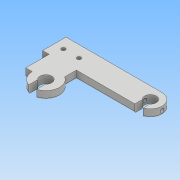
# Autodesk Inventor part: Hand - Digit 0-1
Saved by Autodesk Inventor 2017 (Build 210142000, 142)
## iProperties
Created: 2016-09-27
Part Number: Hand - Digit 0-1
Material: Generic
Document SubType Name: Modeling
Designer: cmcdona
Density: 1 g/cm^3
Appearance: Default
Author: cmcdona
Autodesk Inventor part; units mm, degrees
ref_plane "YZ Plane" through (0, 0, 0) normal (1, 0, 0) x (0, 1, 0)
ref_plane "XZ Plane" through (0, 0, 0) normal (0, 1, 0) x (-1, 0, 0)
sketch "Sketch1" plane through (0, 0, 0) normal (0, 0, 1) x (1, 0, 0)
  line L0 (0, 0) -> (5, 0)
  line L1 (5, 0) -> (5, -18)
  line L2 (5, -18) -> (26, -18)
  line L3 (26, -18) -> (26, 0)
  line L4 (26, 0) -> (74, 0)
  arc A0 (74, 0) -> (74, 18) centre (74, 9) ccw
  line L5 (74, 18) -> (0, 18)
  line L6 (0, 18) -> (0, 0)
  circle A1 centre (20.5, -18) radius 10.5
  dimension "d0" = 5
  dimension "d1" = 18
  dimension "d2" = 21
  dimension "d3" = 18
  dimension "d4" = 48
  dimension "d5" = 18
  dimension "d6" = 9
  dimension "d7" = 74
  dimension "d8" = 21
  constraints: 14 end point, 3 perpendicular, 3 point on line, 2 centre point, 2 horizontal, 2 point on circle
  measures "d0" distance of L0.start L0.end
  measures "d1" distance of L0.end L1.end
  measures "d2" distance of L1.end L2.end
  measures "d3" distance of L2.end L3.end
  measures "d4" distance of L3.end L4.end
  measures "d5" distance of L4.end L5.start
  measures "d6" radius of A0
  measures "d7" distance of L5.start L5.end
  measures "d8" diameter of A1
extrude "Extrusion1" add sketch "Sketch1" along normal blind 6
sketch "Sketch2" plane through (0, 0, 0) normal (0, 0, -1) x (-1, 0, 0)
  circle A0 centre (-74, 9) radius 4.5
  arc A1 (-26, -9.0557) -> (-10, -18) centre (-20.5, -18) ccw projected
  circle A2 centre (-20.5, -18) radius 4.5
  point P0 (0, 0)
  dimension "d11" = 9
  dimension "d12" = 9
  constraints: 2 centre point, 1 coincident
  measures "d11" diameter of A0
  measures "d12" diameter of A2
extrude "Extrusion2" cut sketch "Sketch2" against normal through all
sketch "Sketch3" plane through (0, 0, 0) normal (0, 0, -1) x (-1, 0, 0)
  circle A0 centre (-7, 9) radius 1.5
  circle A1 centre (-19, 9) radius 1.5
  point P0 (0, 0)
  dimension "d16" = 3
  dimension "d17" = 3
  constraints: 2 centre point
  measures "d16" diameter of A0
  measures "d17" diameter of A1
extrude "Extrusion3" cut sketch "Sketch3" against normal through all
ref_plane "Work Plane1" through (83, 0, 0) normal (-1, 0, 0) x (0, 0, 1)
sketch "Sketch4" plane through (83, 0, 0) normal (-1, 0, 0) x (0, 0, 1)
  circle A0 centre (3, 9) radius 1.5
  point P0 (0, 0)
  dimension "d22" = 3
  constraints: 1 centre point
  measures "d22" diameter of A0
extrude "Extrusion4" cut sketch "Sketch4" along normal blind 18
fillet "Fillet3" radius 1 8 edges at (83, 9, 0) (50, 0, 0) (37, 18, 0) (2.5, 0, 0) (5, -9, 0) (25.6235, -27.1652, 0) (7.5, -18, 0) (26, -4.5279, 0)
sketch "Sketch5" plane through (0, 18, 6) normal (0, 1, 0) x (1, 0, 0)
  circle A0 centre (69, 2.5) radius 1.5
  circle A1 centre (58, 2.5) radius 1.5
  point P0 (0, 6)
  dimension "d26" = 3
  dimension "d27" = 3
  constraints: 2 centre point
  measures "d26" diameter of A0
  measures "d27" diameter of A1
extrude "Extrusion5" cut sketch "Sketch5" against normal blind 5
sketch "Sketch6" plane through (0, 0, 6) normal (0, 0, 1) x (1, 0, 0)
  line L0 (71, 0) -> (77, 0)
  line L1 (77, 0) -> (77, 6)
  line L2 (77, 6) -> (71, 6)
  line L3 (71, 6) -> (71, 0)
  line L4 (17.5, -18) -> (23.5, -18)
  line L5 (23.5, -18) -> (23.5, -29)
  line L6 (23.5, -29) -> (17.5, -29)
  line L7 (17.5, -29) -> (17.5, -18)
  point P0 (0, 0)
  dimension "d30" = 6
  dimension "d31" = 6
  dimension "d32" = 6
  dimension "d33" = 11
  constraints: 16 end point, 4 parallel, 2 horizontal, 2 perpendicular
  measures "d30" distance of L2.end L1.end
  measures "d31" distance of L1.end L0.end
  measures "d32" distance of L5.end L6.end
  measures "d33" distance of L4.end L5.end
extrude "Extrusion6" cut sketch "Sketch6" against normal through all
body "Solid1"
